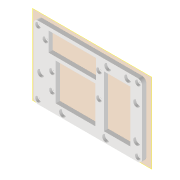
# Autodesk Inventor part: 11_Wellplatespacer_magnetic
Saved by Autodesk Inventor 2022.5 (Build 265521000, 521)
## iProperties
Created: 2023-01-07
Part Number: 11_Wellplatespacer_magnetic
Material: Generisch
Document SubType Name: Modeling
Designer: diederichbenedict
Density: 1 g/cm^3
Appearance: Vorgabe
Author: diederichbenedict
Autodesk Inventor part; units mm, degrees
ref_plane "YZ Plane" through (0, 0, 0) normal (1, 0, 0) x (0, 1, 0)
ref_plane "XZ Plane" through (0, 0, 0) normal (0, 1, 0) x (-1, 0, 0)
ref_plane "Arbeitsebene1" through (0, 0, 0) normal (0, 0, 1) x (1, 0, 0)
sketch "Skizze1" plane through (0, 0, 0) normal (0, 0, 1) x (1, 0, 0)
  line L0 (8.6, 2.25) -> (8.6, -41.35) projected
  line L1 (8.6, -41.35) -> (-37.9, -41.35) projected
  line L2 (-37.9, -41.35) -> (-37.9, 2.25) projected
  line L3 (-37.9, 2.25) -> (8.6, 2.25) projected
  line L4 (9.6, 6.25) -> (-46.4, 6.25) projected
  line L5 (-46.4, 32.25) -> (-46.4, 6.25) projected
  line L6 (9.6, 32.25) -> (-46.4, 32.25) projected
  line L7 (9.6, 6.25) -> (9.6, 32.25) projected
  circle A0 centre (13.1, -11.2637) radius 1.4 projected
  circle A1 centre (-42.4, -11.2637) radius 1.4 projected
  circle A2 centre (-42.4, -31.25) radius 1.4 projected
  line L8 (18.9, -41.35) -> (18.9, 19.75) projected
  line L9 (18.9, 19.75) -> (58.9, 19.75) projected
  line L10 (58.9, 19.75) -> (58.9, 19.25) projected
  line L11 (58.9, 19.25) -> (55.9, 19.25) projected
  line L12 (55.9, 17.6031) -> (55.9, 19.25) projected
  line L13 (63.9, 17.6031) -> (55.9, 17.6031) projected
  line L14 (63.9, 27.75) -> (63.9, 17.6031) projected
  arc A3 (63.9, 27.75) -> (58.9, 32.75) centre (58.9, 27.75) ccw projected
  line L15 (58.9, 32.75) -> (-58.9, 32.75) projected
  arc A4 (-58.9, 32.75) -> (-63.9, 27.75) centre (-58.9, 27.75) ccw projected
  line L16 (-63.9, -47.75) -> (-63.9, 27.75) projected
  arc A5 (-63.9, -47.75) -> (-58.9, -52.75) centre (-58.9, -47.75) ccw projected
  line L17 (-58.9, -52.75) -> (58.9, -52.75) projected
  arc A6 (58.9, -52.75) -> (63.9, -47.75) centre (58.9, -47.75) ccw projected
  line L18 (63.9, -47.75) -> (63.9, 0.8969) projected
  line L19 (55.9, 0.8969) -> (63.9, 0.8969) projected
  line L20 (55.9, -0.75) -> (55.9, 0.8969) projected
  line L21 (58.9, -0.75) -> (55.9, -0.75) projected
  line L22 (58.9, -0.75) -> (58.9, -1.25) projected
  line L23 (58.9, -1.25) -> (49.9, -1.25) projected
  line L24 (49.9, -1.25) -> (49.9, -41.35) projected
  line L25 (49.9, -41.35) -> (18.9, -41.35) projected
  circle A7 centre (13.1, 17.25) radius 1.4 projected
  circle A8 centre (-50.2191, 17.25) radius 1.4 projected
  line L26 (63.9, 17.6031) -> (63.9, 0.8969)
  line L27 (49.9, -1.25) -> (49.9, 19.75)
  line L28 (18.9, 6.25) -> (9.6, 6.25)
  line L29 (9.6, 6.25) -> (9.6, 2.25)
  line L30 (9.6, 2.25) -> (8.6, 2.25)
  line L31 (-37.9, 2.25) -> (-46.4, 2.25)
  line L32 (-46.4, 2.25) -> (-46.4, 6.25)
  line L33 (9.6, 32.25) -> (9.6, 32.75)
  line L34 (-46.4, 32.25) -> (-46.4, 32.75)
  circle A9 centre (58.9, 27.75) radius 1.4
  circle A10 centre (58.9, -47.75) radius 1.4
  circle A11 centre (-58.9, -47.75) radius 1.4
  circle A12 centre (-58.9, 27.75) radius 1.4
  line L35 (-46.4, 32.75) -> (9.6, 32.75)
  line L36 (9.6, 32.75) -> (9.6, 28.75)
  line L37 (9.6, 28.75) -> (-46.4, 28.75)
  line L38 (-46.4, 28.75) -> (-46.4, 32.75)
  point P0 (0, 0)
  point P1 (-46.4, 28.75)
  dimension "d0" = 2.8
  dimension "d1" = 2.8
  dimension "d2" = 2.8
  dimension "d3" = 2.8
  dimension "d29" = 4
  constraints: 26 end point, 8 point on line, 4 centre point, 4 coincident, 4 perpendicular, 3 parallel, 2 vertical, 1 horizontal
  measures "d0" diameter of A9
  measures "d1" diameter of A10
  measures "d2" diameter of A11
  measures "d3" diameter of A12
  measures "d29" distance of L35.end L36.end
extrude "Extrusion1" add sketch "Skizze1" along normal blind 5 contours L30 L29 L28 L8 L25 L24 L23 L22 L21 L20 L19 L18 A6 L17 A5 L16 A4 L15 L34 L5 L32 L31 L2 L1 L0 | L3 L31 L32 L4 L29 L30 | L7 L33 L15 A3 L14 L13 L12 L11 L10 L9 L8 L28 | L37 L5 L6 L7 | L6 L34 L15 L33 | L9 L10 L11 L12 L13 L26 L19 L20 L21 L22 L23 L27
sketch "Skizze3" plane through (0, 0, 5) normal (0, 0, 1) x (1, 0, 0)
  line L0 (-58.9, -52.75) -> (58.9, -52.75) projected
  arc A0 (58.9, -52.75) -> (63.9, -47.75) centre (58.9, -47.75) ccw projected
  line L1 (63.9, -47.75) -> (63.9, 27.75) projected
  arc A1 (63.9, 27.75) -> (58.9, 32.75) centre (58.9, 27.75) ccw projected
  line L2 (58.9, 32.75) -> (-58.9, 32.75) projected
  line L3 (9.6, 28.75) -> (9.6, 6.25) projected
  line L4 (9.6, 6.25) -> (-46.4, 6.25) projected
  line L5 (-46.4, 6.25) -> (-46.4, 28.75) projected
  arc A2 (-58.9, 32.75) -> (-63.9, 27.75) centre (-58.9, 27.75) ccw projected
  line L6 (-63.9, 27.75) -> (-63.9, -47.75) projected
  arc A3 (-63.9, -47.75) -> (-58.9, -52.75) centre (-58.9, -47.75) ccw projected
  circle A4 centre (13.1, 17.25) radius 1.4 projected
  circle A5 centre (58.9, 27.75) radius 1.4 projected
  circle A6 centre (13.1, -11.2637) radius 1.4 projected
  circle A7 centre (-42.4, -11.2637) radius 1.4 projected
  circle A8 centre (-42.4, -31.25) radius 1.4 projected
  circle A9 centre (-50.2191, 17.25) radius 1.4 projected
  circle A10 centre (-58.9, 27.75) radius 1.4 projected
  circle A11 centre (-58.9, -47.75) radius 1.4 projected
  circle A12 centre (58.9, -47.75) radius 1.4 projected
  line L7 (8.6, 2.25) -> (8.6, -41.35) projected
  line L8 (8.6, -41.35) -> (-37.9, -41.35) projected
  line L9 (-37.9, -41.35) -> (-37.9, 2.25) projected
  line L10 (-37.9, 2.25) -> (8.6, 2.25) projected
  line L11 (18.9, -41.35) -> (18.9, 19.75) projected
  line L12 (18.9, 19.75) -> (49.9, 19.75) projected
  line L13 (49.9, 19.75) -> (49.9, -41.35) projected
  line L14 (49.9, -41.35) -> (18.9, -41.35) projected
  line L15 (-46.4, 28.75) -> (9.6, 28.75) projected
  point P0 (0, 0)
hole "Bohrung1" at (58.9, -47.75, 5) at (-58.9, -47.75, 5) at (-42.4, -31.25, 5) at (-42.4, -11.2637, 5) at (-50.2191, 17.25, 5) at (-58.9, 27.75, 5) at (13.1, -11.2637, 5) at (13.1, 17.25, 5) at (58.9, 27.75, 5) direction (0, 0, -1) diameter 2.9 end through all counterbore diameter 6.5 counterbore depth 3
ref_plane "Arbeitsebene2" through (55.9, -6.9963, -17.125) normal (-1, 0, 0) x (0, 0, 1)
sketch "Skizze7" plane through (0, 0, 5) normal (0, 0, 1) x (1, 0, 0)
  circle A0 centre (13.1, -11.2637) radius 3.25 projected
  line L0 (18.9, -41.35) -> (18.9, 19.75) projected
  line L1 (18.9, 19.75) -> (49.9, 19.75) projected
  line L2 (49.9, 19.75) -> (49.9, -41.35) projected
  line L3 (49.9, -41.35) -> (18.9, -41.35) projected
  line L4 (-37.9, -41.35) -> (-37.9, 2.25) projected
  line L5 (-37.9, 2.25) -> (8.6, 2.25) projected
  line L6 (8.6, 2.25) -> (8.6, -41.35) projected
  circle A1 centre (13.1, 17.25) radius 3.25 projected
  circle A2 centre (-58.9, 27.75) radius 3.25 projected
  circle A3 centre (-42.4, -11.2637) radius 3.25 projected
  circle A4 centre (-58.9, -47.75) radius 3.25 projected
  circle A5 centre (58.9, -47.75) radius 3.25 projected
  circle A6 centre (-42.4, -31.25) radius 3.25 projected
  circle A7 centre (-50.2191, 17.25) radius 3.25 projected
  circle A8 centre (58.9, 27.75) radius 3.25 projected
  line L7 (58.9, 32.75) -> (-58.9, 32.75) projected
  arc A9 (-58.9, 32.75) -> (-63.9, 27.75) centre (-58.9, 27.75) ccw projected
  line L8 (-63.9, 27.75) -> (-63.9, -47.75) projected
  arc A10 (-63.9, -47.75) -> (-58.9, -52.75) centre (-58.9, -47.75) ccw projected
  line L9 (-58.9, -52.75) -> (58.9, -52.75) projected
  arc A11 (58.9, -52.75) -> (63.9, -47.75) centre (58.9, -47.75) ccw projected
  line L10 (63.9, -47.75) -> (63.9, 27.75) projected
  arc A12 (63.9, 27.75) -> (58.9, 32.75) centre (58.9, 27.75) ccw projected
  line L11 (9.6, 28.75) -> (9.6, 6.25) projected
  line L12 (9.6, 6.25) -> (-46.4, 6.25) projected
  line L13 (-46.4, 6.25) -> (-46.4, 28.75) projected
  line L14 (-46.4, 28.75) -> (9.6, 28.75) projected
  circle A13 centre (23.4151, 26.1333) radius 4
  circle A14 centre (46.9172, 26.1333) radius 4
  circle A15 centre (57.5383, 6.25) radius 4
  circle A16 centre (57.5383, -32.848) radius 4
  circle A17 centre (20.9293, -47.75) radius 4
  circle A18 centre (-29.9166, -47.75) radius 4
  circle A19 centre (-55.65, -19.55) radius 4
  line L15 (8.6, -41.35) -> (-37.9, -41.35) projected
  point P0 (0, 0)
  dimension "d33" = 8
  dimension "d34" = 8
  dimension "d35" = 8
  dimension "d36" = 8
  dimension "d37" = 8
  dimension "d38" = 8
  dimension "d39" = 8
  constraints: 7 centre point
  measures "d33" diameter of A13
  measures "d34" diameter of A14
  measures "d35" diameter of A15
  measures "d36" diameter of A16
  measures "d37" diameter of A17
  measures "d38" diameter of A18
  measures "d39" diameter of A19
extrude "Extrusion6" cut sketch "Skizze7" against normal blind 3.2 contours A13 | A14 | A15 | A16 | A17 | A18 | A19
